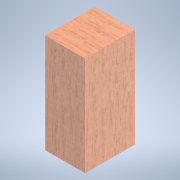
# Autodesk Inventor part: square peg
Saved by Autodesk Inventor 2021 (Build 250183000, 183)
## iProperties
Created: 2020-05-07
Part Number: square peg
Material: Wood (Oak)
Document SubType Name: Modeling
Designer: david
Density: 0.76 g/cm^3
Appearance: White Oak - Natural Medium Gloss
Author: david
Autodesk Inventor part; units mm, degrees
ref_plane "YZ Plane" through (0, 0, 0) normal (1, 0, 0) x (0, 1, 0)
ref_plane "XZ Plane" through (0, 0, 0) normal (0, 1, 0) x (-1, 0, 0)
ref_plane "XY Plane" through (0, 0, 0) normal (0, 0, 1) x (1, 0, 0)
sketch "Sketch1" plane through (0, 0, 0) normal (0, 1, 0) x (-1, 0, 0)
  line L0 (69.0145, -70.0171) -> (28.3745, -70.0171)
  line L1 (28.3745, -70.0171) -> (28.3745, -120.8171)
  line L2 (28.3745, -120.8171) -> (69.0145, -120.8171)
  line L3 (69.0145, -120.8171) -> (69.0145, -70.0171)
  point P0 (0, 0)
  dimension "d0" = 50.8
  dimension "d1" = 40.64
  constraints: 8 end point, 2 parallel, 1 horizontal, 1 perpendicular
  measures "d0" distance of L2.end L0.start
  measures "d1" distance of L1.end L2.end
extrude "Extrusion1" add sketch "Sketch1" along normal blind 101.6
body "Solid1"
